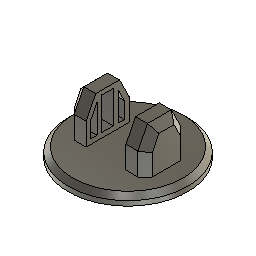
base_top (Autodesk Fusion 360 design; units mm, degrees)
Autodesk Fusion 360 part; units mm, degrees
sketch "Sketch1" plane through (0, 0, 0) normal (0, 0, 1) x (1, 0, 0)
  circle A0 centre (0, 0) radius 62.5
  line L0 (-11, 29) -> (11, 29)
  line L1 (11, -29) -> (-11, -29)
  line L2 (-11, 29) -> (11, -29) construction
  line L3 (11, 29) -> (-11, -29) construction
  line L4 (11, 29) -> (11, -29)
  line L5 (-11, -29) -> (-11, 29)
  circle A1 centre (0, 0) radius 35
  circle A2 centre (0, 0) radius 6.35
  dimension "d1" = 22
  dimension "d2" = 58
  dimension "d3" = 70
  dimension "d19" = 12.7
  constraint horizontal L0
  constraint perpendicular L0 L4
  constraint parallel L0 L1
  constraint parallel L4 L5
  constraint coincident A0.centre L2
  constraint coincident A0.centre L3
  constraint coincident A0.centre A1.centre
  measures "d1" distance of L1.start L1.end
  measures "d2" distance of L0.end L1.start
  measures "d3" diameter of A1
  measures "d19" diameter of A2
extrude "Extrude1" add sketch "Sketch1" along normal blind 10 contours A0 | L0 L1 L4 L5 | A1 | A2 makes body 1
ref_plane "WorkPlane1" through (13.4, 0, 0) normal (1, 0, 0) x (0, 1, 0)
sketch "Sketch2" plane through (13.4, 0, 0) normal (1, 0, 0) x (0, 1, 0)
  line L0 (-6, 15) -> (6, 15)
  line L1 (6, 15) -> (6, 49)
  line L2 (6, 49) -> (-6, 49)
  line L3 (-6, 49) -> (-6, 15)
  line L4 (0, 49) -> (0, 15) construction
  line L5 (-22.5, 9.9405) -> (-22.5, 33.5)
  line L6 (-12.5, 53.5) -> (12.5, 53.5)
  line L7 (22.5, 33.5) -> (22.5, 9.9405)
  line L8 (-22.5, 9.9405) -> (22.5, 9.9405)
  line L9 (12.5, 53.5) -> (22.5, 33.5)
  line L10 (-12.5, 53.5) -> (-22.5, 33.5)
  dimension "d7" = 12
  dimension "d8" = 34
  constraint horizontal L0
  constraint vertical L1
  constraint horizontal L2
  constraint vertical L3
  constraint midpoint L2 L4.start
  constraint midpoint L0 L4.end
  constraint parallel L5 L7
  constraint perpendicular L7 L8
  constraint symmetric L4 L6.end L6.start
  constraint symmetric L4 L7.start L5.end
  measures "d7" distance of L0.start L0.end
  measures "d8" distance of L0.start L2.end
extrude "Extrude2" add sketch "Sketch2" along normal blind 20 separate body contours L0 L1 L2 L3 | L5 L6 L7 L8 L9 L10 makes body 2
extrude "Extrude3" cut sketch "Sketch2" along normal blind 40 contours L0 L1 L2 L3 bodies 2
mirror "Mirror1" about plane through (0, 0, 0) normal (1, 0, 0) of bodies 2 makes body 3
extrude "Extrude4" cut sketch "Sketch1" along normal blind 4 contours A2 bodies 1
shell "Shell1" thickness 5 removed faces 2 at (13.4, -11.5, 32.5) at (-13.4, -11.5, 32.5) on bodies 2 3
extrude "Extrude5" add 1 faces at (20.0667, -2, 15) along direction (0, 0, 1) blind 35 on bodies 2 bodies 2
sketch "Sketch3" plane through (13.4, 0, 0) normal (-1, 0, 0) x (0, -1, 0)
  line L0 (12.5, 53.5) -> (-12.5, 53.5)
  line L1 (-12.5, 53.5) -> (-22.5, 33.5)
  line L2 (-22.5, 33.5) -> (-22.5, 9.9405)
  line L3 (-22.5, 9.9405) -> (22.5, 9.9405)
  line L4 (22.5, 9.9405) -> (22.5, 33.5)
  line L5 (22.5, 33.5) -> (12.5, 53.5)
  line L6 (17.5, 14.9405) -> (11, 14.9405)
  line L7 (11, 14.9405) -> (11, 45.3197)
  line L8 (11, 45.3197) -> (17.5, 32.3197)
  line L9 (17.5, 32.3197) -> (17.5, 14.9405)
  line L10 (-17.5, 32.3197) -> (-11, 45.3197)
  line L11 (-11, 45.3197) -> (-11, 14.9405)
  line L12 (-11, 14.9405) -> (-17.5, 14.9405)
  line L13 (-17.5, 14.9405) -> (-17.5, 32.3197)
  line L14 (-11, 45.3197) -> (11, 45.3197)
  line L15 (11, 45.3197) -> (11, 14.9405)
  line L16 (11, 14.9405) -> (-11, 14.9405)
  line L17 (-11, 14.9405) -> (-11, 45.3197)
  circle A0 centre (0, 37.4301) radius 2
  dimension "d25" = 4
  constraint horizontal L14
  constraint vertical L15
  constraint horizontal L16
  constraint vertical L17
  constraint coincident L6.end L7.start
  constraint coincident L10.end L11.start
  measures "d25" diameter of A0
extrude "Extrude6" add sketch "Sketch3" along normal blind 4.25 contours A0 bodies 2
move_body "Move1" bodies 3 to x (1, 0, 0) y (0, 1, 0) z (0, 0, 1) at (-5, 0, 0)
move_body "Move2" bodies 2 to x (1, 0, 0) y (0, 1, 0) z (0, 0, 1) at (4, 0, 0)
move_body "Move4" bodies 2 to x (1, 0, 0) y (0, 1, 0) z (0, 0, 1) at (3, 0, 0)
move_body "Move5" bodies 3 to x (1, 0, 0) y (0, 1, 0) z (0, 0, 1) at (-3, 0, 0)
chamfer "Chamfer1" distance 5 angle 45 1 edges at (-58.2705, -22.601, 10) on bodies 1
chamfer "Chamfer2" distance 7.5 angle 45 10 edges at (40.4, 0, 53.5) (40.4, -17.5, 43.5) (40.4, 17.5, 43.5) (40.4, 22.5, 21.7203) (40.4, -22.5, 21.7203) (-41.4, 0, 53.5) (-41.4, -17.5, 43.5) (-41.4, -22.5, 21.7203) (-41.4, 17.5, 43.5) (-41.4, 22.5, 21.7203) on bodies 2 3
